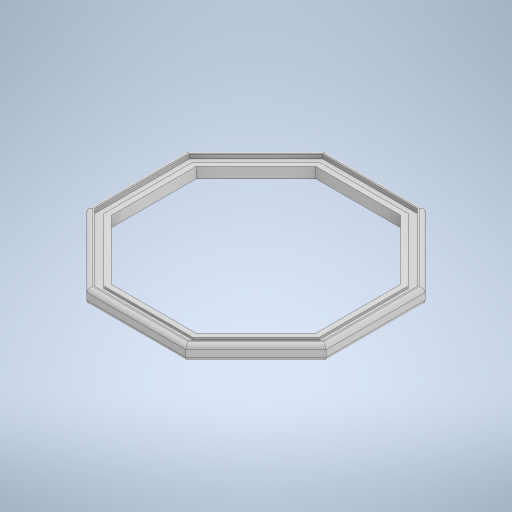
# Autodesk Inventor part: OV-PAM_ring_2
Saved by Autodesk Inventor 2024 (Build 280153000, 153)
## iProperties
Created: 2023-06-19
Part Number: OV-PAM_ring_2
Material: 일반
Document SubType Name: Modeling
Designer: jsw
Density: 1 g/cm^3
Appearance: 기본값
Author: jsw
Autodesk Inventor part; units mm, degrees
ref_plane "YZ Plane" through (0, 0, 0) normal (1, 0, 0) x (0, 1, 0)
ref_plane "XZ Plane" through (0, 0, 0) normal (0, 1, 0) x (-1, 0, 0)
sketch "스케치1" plane through (0, 0, 0) normal (0, 1, 0) x (-1, 0, 0)
  line L0 (-32.5919, 13.5) -> (-13.5, 32.5919)
  line L1 (-13.5, 32.5919) -> (13.5, 32.5919)
  line L2 (13.5, 32.5919) -> (32.5919, 13.5)
  line L3 (32.5919, 13.5) -> (32.5919, -13.5)
  line L4 (32.5919, -13.5) -> (13.5, -32.5919)
  line L5 (13.5, -32.5919) -> (-13.5, -32.5919)
  line L6 (-13.5, -32.5919) -> (-32.5919, -13.5)
  line L7 (-32.5919, -13.5) -> (-32.5919, 13.5)
  line L8 (35.7919, 14.8255) -> (35.7919, -14.8255)
  line L9 (35.7919, -14.8255) -> (14.8255, -35.7919)
  line L10 (14.8255, -35.7919) -> (-14.8255, -35.7919)
  line L11 (-14.8255, -35.7919) -> (-35.7919, -14.8255)
  line L12 (-35.7919, -14.8255) -> (-35.7919, 14.8255)
  line L13 (-35.7919, 14.8255) -> (-14.8255, 35.7919)
  line L14 (-14.8255, 35.7919) -> (14.8255, 35.7919)
  line L15 (14.8255, 35.7919) -> (35.7919, 14.8255)
  point P0 (0, 0)
  point P1 (0, 0)
  point P2 (0, 0)
  dimension "d0" = 27
  dimension "d1" = 3.2
  constraints: 32 end point, 2 coincident, 2 horizontal, 34 other
  measures "d0" distance of L2.end L3.end
  measures "d1" distance between parallel lines of L8 L3
extrude "돌출1" add sketch "스케치1" along normal blind 4.4 contours L0 L1 L2 L3 L4 L5 L6 L7 | L8 L9 L10 L11 L12 L13 L14 L15
sketch "스케치3" plane through (0, 0, 0) normal (0, -1, 0) x (1, 0, 0)
  line L0 (-13.3343, 32.1919) -> (13.3343, 32.1919)
  line L1 (13.3343, 32.1919) -> (32.1919, 13.3343)
  line L2 (32.1919, 13.3343) -> (32.1919, -13.3343)
  line L3 (32.1919, -13.3343) -> (13.3343, -32.1919)
  line L4 (13.3343, -32.1919) -> (-13.3343, -32.1919)
  line L5 (-13.3343, -32.1919) -> (-32.1919, -13.3343)
  line L6 (-32.1919, -13.3343) -> (-32.1919, 13.3343)
  line L7 (-32.1919, 13.3343) -> (-13.3343, 32.1919)
  line L8 (-14.1627, 34.1919) -> (14.1627, 34.1919)
  line L9 (14.1627, 34.1919) -> (34.1919, 14.1627)
  line L10 (34.1919, 14.1627) -> (34.1919, -14.1627)
  line L11 (34.1919, -14.1627) -> (14.1627, -34.1919)
  line L12 (14.1627, -34.1919) -> (-14.1627, -34.1919)
  line L13 (-14.1627, -34.1919) -> (-34.1919, -14.1627)
  line L14 (-34.1919, -14.1627) -> (-34.1919, 14.1627)
  line L15 (-34.1919, 14.1627) -> (-14.1627, 34.1919)
  line L16 (-14.8255, 35.7919) -> (14.8255, 35.7919) projected
  point P0 (0, 0)
  point P1 (0, 0)
  point P2 (0, 0)
  point P3 (0, 0)
  dimension "d9" = 2
  dimension "d144" = 1.6
  constraints: 32 end point, 3 coincident, 2 horizontal, 34 other
  measures "d9" distance between parallel lines of L8 L0
  measures "d144" distance between parallel lines of L16 L8
extrude "돌출3" cut sketch "스케치3" against normal blind 1.2
sketch "스케치14" plane through (0, 0, 0) normal (0, -1, 0) x (1, 0, 0)
  line L0 (32.1919, 13.3343) -> (13.3343, 32.1919) projected
  line L1 (13.3343, 32.1919) -> (-13.3343, 32.1919) projected
  line L2 (-13.3343, 32.1919) -> (-32.1919, 13.3343) projected
  line L3 (-32.1919, 13.3343) -> (-32.1919, -13.3343) projected
  line L4 (-32.1919, -13.3343) -> (-13.3343, -32.1919) projected
  line L5 (-13.3343, -32.1919) -> (13.3343, -32.1919) projected
  line L6 (13.3343, -32.1919) -> (32.1919, -13.3343) projected
  line L7 (32.1919, -13.3343) -> (32.1919, 13.3343) projected
  point P0 (0, 0)
extrude "돌출16" cut sketch "스케치14" against normal blind 0.6
sketch "스케치15" plane through (0, 0.6, 0) normal (0, -1, 0) x (1, 0, 0)
  line L0 (-12.6716, 30.5919) -> (12.6716, 30.5919)
  line L1 (12.6716, 30.5919) -> (30.5919, 12.6716)
  line L2 (30.5919, 12.6716) -> (30.5919, -12.6716)
  line L3 (30.5919, -12.6716) -> (12.6716, -30.5919)
  line L4 (12.6716, -30.5919) -> (-12.6716, -30.5919)
  line L5 (-12.6716, -30.5919) -> (-30.5919, -12.6716)
  line L6 (-30.5919, -12.6716) -> (-30.5919, 12.6716)
  line L7 (-30.5919, 12.6716) -> (-12.6716, 30.5919)
  line L8 (-13.3343, 32.1919) -> (13.3343, 32.1919) projected
  point P0 (0, 0)
  point P1 (0, 0)
  dimension "d140" = 1.6
  constraints: 16 end point, 1 coincident, 1 horizontal, 17 other
  measures "d140" distance between parallel lines of L0 L8
extrude "돌출17" cut sketch "스케치15" against normal up to surface (3.8 mm away)
ref_plane "작업 평면3" through (0, 2.2, 0) normal (0, -1, 0) x (1, 0, 0)
mirror "미러6" about plane through (0, 2.2, 0) normal (0, -1, 0) of "돌출3", "돌출16"
fillet "모깎기2" radius 1.2 16 edges at (0, 0, 35.7919) (-25.3087, 0, 25.3087) (-35.7919, 0, 0) (-25.3087, 0, -25.3087) (0, 0, -35.7919) (25.3087, 0, -25.3087) (35.7919, 0, 0) (25.3087, 0, 25.3087) (-25.3087, 4.4, 25.3087) (-35.7919, 4.4, 0) (-25.3087, 4.4, -25.3087) (0, 4.4, -35.7919) (25.3087, 4.4, -25.3087) (35.7919, 4.4, 0) (25.3087, 4.4, 25.3087) (0, 4.4, 35.7919)
